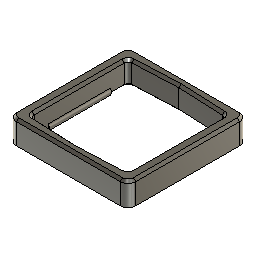
datanectics keyboard switch shackle_v7 (Autodesk Fusion 360 design; units mm, degrees)
Autodesk Fusion 360 part; units mm, degrees
note: some values were not read from the file. Chosen so that the rebuilt part matches the saved one: which pieces of a blend or face edit are solid.
sketch "Sketch1" plane through (0, 0, 0) normal (0, 0, 1) x (1, 0, 0)
  line L0 (0, 18.188074) -> (0, -15.507009) construction
  line L1 (-13.782609, 0) -> (15.781677, 0) construction
  line L2 (6.295, 6.295) -> (-6.295, 6.295) construction
  line L3 (-6.295, 6.295) -> (-6.295, -6.295)
  line L4 (-6.295, -6.295) -> (6.295, -6.295) construction
  line L5 (6.295, -6.295) -> (6.295, 6.295)
  line L6 (6.295, 6.295) -> (-6.295, -6.295) construction
  line L7 (-6.295, 6.295) -> (6.295, -6.295) construction
  line L8 (-6.295, 6.295) -> (0, 6.575)
  line L9 (6.295, 6.295) -> (0, 6.575)
  line L10 (6.295, -6.295) -> (0, -6.575)
  line L11 (-6.295, -6.295) -> (0, -6.575)
  arc A0 (-5.817218, 6.316252) -> (-6.295, 5.816746) centre (-5.795, 5.816746) ccw
  arc A1 (-6.295, -5.816746) -> (-5.817218, -6.316252) centre (-5.795, -5.816746) ccw
  arc A2 (5.817218, -6.316252) -> (6.295, -5.816746) centre (5.795, -5.816746) ccw
  arc A3 (6.295, 5.816746) -> (5.817218, 6.316252) centre (5.795, 5.816746) ccw
  line L12 (-7.695, 7.695) -> (-7.695, -7.695)
  line L13 (-7.695, -7.695) -> (7.695, -7.695)
  line L14 (7.695, -7.695) -> (7.695, 7.695)
  line L15 (7.695, 7.695) -> (-7.695, 7.695)
  dimension "d8" = 12.59
  dimension "d9" = 12.59
  dimension "d10" = 0.28
  dimension "d11" = 0.5
  dimension "d12" = 0.5
  dimension "d13" = 1.4
  constraint coincident origin L1
  constraint perpendicular L0 L1
  constraint vertical L0
  constraint horizontal L2
  constraint perpendicular L2 L3
  constraint parallel L2 L4
  constraint parallel L3 L5
  constraint coincident L6 origin
  constraint coincident L7 origin
  constraint coincident L0 L8.end
  constraint coincident L0 origin
  constraint symmetric L1 L2.start L4.end
  constraint symmetric L1 L2.end L3.end
  constraint symmetric L1 L8.end L10.end
  constraint tangent L8 A0
  constraint tangent L3 A0
  constraint tangent L3 A1
  constraint tangent L11 A1
  constraint symmetric L0 A0 A3
  constraint symmetric L0 A1 A2
  measures "d8" distance of L3.end L4.end
  measures "d9" distance of L2.end L3.end
  measures "d10" distance of L2 L8.end
  measures "d11" radius of A0
  measures "d12" radius of A1
extrude "Extrude1" add sketch "Sketch1" along normal blind 3 contours L3 L8 A0 | L3 L11 A1 | L5 L9 A3 | L5 L10 A2 | L12 L13 L14 L15 picked at (-6.201969, 6.206015) picked at (-6.201969, -6.206015) picked at (6.201969, 6.206015) picked at (6.201969, -6.206015) picked at (7.228333, 1.938915)
sketch "Sketch3" plane through (0, 0, 0) normal (0, 1, 0) x (1, 0, 0)
  line L0 (6.295, 0) -> (6.295, -3)
  line L1 (6.295, -3) -> (6.295, 0)
  line L2 (-6.295, 0) -> (-6.295, -3)
  line L3 (-6.295, -3) -> (-6.295, 0)
  arc A0 (6.295, 0) -> (6.295, -0.8) centre (6.742214, -0.4) ccw
  line L4 (0, -4.785635) -> (0, 3.559368) construction
  arc A1 (-6.295, -0.8) -> (-6.295, 0) centre (-6.742214, -0.4) ccw
  dimension "d16" = 0.8
  dimension "d17" = 0.6
  constraint coincident L0 A0.end
  constraint coincident L0.start L1.end
  constraint vertical L4
  constraint coincident origin L4
  constraint symmetric L0.start L4 L2.start
  constraint symmetric A0.end L4 A1.start
  constraint symmetric A0 L4 A1
  measures "d16" distance of L0.start A0.end
  measures "d17" radius of A0
extrude "Extrude2" add sketch "Sketch3" along normal mid plane 8
fillet "Fillet2" radius 1 4 edges at (7.695, -7.695, 1.5) (7.695, 7.695, 1.5) (-7.695, 7.695, 1.5) (-7.695, -7.695, 1.5)
chamfer "Chamfer1" distance 0.3 angle 45 12 edges at (2.908609, 6.445626, 0) (6.156323, 6.162354, 0) (6.295, 4.908373, 0) (-2.908609, 6.445626, 0) (-6.295, 4.908373, 0) (-6.156323, 6.162354, 0) (-2.908609, -6.445626, 0) (-6.156323, -6.162354, 0) (-6.295, -4.908373, 0) (2.908609, -6.445626, 0) (6.295, -4.908373, 0) (6.156323, -6.162354, 0)
chamfer "Chamfer2" distance 0.3 angle 45 1 faces at (7.228333, 1.938915, 3)
equation "d9 = d8"
